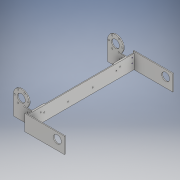
# Autodesk Inventor part: Pivot Bracket 2
Saved by Autodesk Inventor 2017 (Build 210142000, 142)
## iProperties
Created: 2017-06-10
Part Number: Pivot Bracket 2
Material: Generic
Document SubType Name: Modeling
Designer: Matthew
Density: 1 g/cm^3
Appearance: Aluminum - Polished
Author: Matthew
Autodesk Inventor part; units mm, degrees
ref_plane "YZ Plane" through (0, 0, 0) normal (1, 0, 0) x (0, 1, 0)
ref_plane "XZ Plane" through (0, 0, 0) normal (0, 1, 0) x (-1, 0, 0)
ref_plane "XY Plane" through (0, 0, 0) normal (0, 0, 1) x (1, 0, 0)
sketch "Sketch1" plane through (0, 0, 0) normal (0, 1, 0) x (-1, 0, 0)
  line L0 (0, 0) -> (-88.9, 0)
  line L1 (-88.9, 0) -> (-88.9, -3.175)
  line L2 (-88.9, -3.175) -> (0, -3.175)
  line L3 (0, -3.175) -> (0, 0)
  dimension "d0" = 88.9
  dimension "d1" = 3.175
  constraints: 8 end point, 2 parallel, 1 horizontal, 1 perpendicular
  measures "d0" distance of L2.end L1.end
  measures "d1" distance of L1.end L0.end
extrude "Extrusion1" add sketch "Sketch1" along normal blind 25.4
sketch "Sketch2" plane through (0, 0, 0) normal (0, 0, 1) x (1, 0, 0)
  line L0 (88.9, 0) -> (88.9, 25.4) projected
  circle A0 centre (88.9, 12.7) radius 3.175
  point P0 (0, 0)
  dimension "d4" = 6.35
  constraints: 1 centre point, 1 midpoint
  measures "d4" diameter of A0
extrude "Extrusion2" cut sketch "Sketch2" against normal blind 25.4
sketch "Sketch3" plane through (0, 0, 0) normal (0, 0, 1) x (1, 0, 0)
  arc A0 (88.9, 15.875) -> (88.9, 9.525) centre (88.9, 12.7) ccw projected
  line L0 (88.9, 25.4) -> (0, 25.4) projected
  circle A1 centre (88.9, 12.7) radius 12.7
  line L1 (88.9, 15.875) -> (88.9, 25.4) projected
  circle A2 centre (88.9, 12.7) radius 3.175
  point P0 (0, 0)
  constraints: 2 coincident, 2 vertical alignment, 4 other
extrude "Extrusion3" add sketch "Sketch3" against normal blind 3.175
sketch "Sketch4" plane through (0, 0, -3.175) normal (-1, 0, 0) x (0, 0, 1)
  line L0 (0, 0) -> (0, 25.4) projected
  line L1 (0, 0) -> (53.975, 0)
  line L2 (53.975, 0) -> (53.975, 25.4)
  line L3 (53.975, 25.4) -> (0, 25.4)
  line L4 (0, 25.4) -> (0, 0)
  point P0 (3.175, 0)
  dimension "d9" = 53.975
  constraints: 8 end point, 2 parallel, 1 horizontal, 1 perpendicular
  measures "d9" distance of L3.end L2.end
extrude "Extrusion4" add sketch "Sketch4" against normal blind 3.175
sketch "Sketch5" plane through (3.175, 0, -3.175) normal (1, 0, 0) x (0, 0, -1)
  line L0 (-3.175, 25.4) -> (-53.975, 25.4) projected
  line L1 (-3.175, 25.4) -> (-53.975, 12.7)
  line L2 (-53.975, 12.7) -> (-53.975, -12.7)
  line L3 (-53.975, 25.4) -> (-53.975, 0) projected
  line L4 (-53.975, -12.7) -> (-3.175, 0)
  line L5 (-3.175, 25.4) -> (-3.175, 0) projected
  line L6 (-3.175, 25.4) -> (-3.175, 0)
  dimension "d12" = 12.7
  dimension "d13" = 25.4
  constraints: 8 end point, 3 equal length, 1 point on line, 1 vertical alignment
  measures "d12" distance of L0.end L1.end
  measures "d13" distance of L1.end L2.end
sketch "Sketch6" plane through (3.175, 0, -3.175) normal (1, 0, 0) x (0, 0, -1)
  line L0 (-3.175, 25.4) -> (-3.175, 0) projected
  line L1 (-3.175, 25.4) -> (-53.975, 25.4) projected
  line L2 (-53.975, 25.4) -> (-53.975, 0) projected
  line L3 (-53.975, 0) -> (-3.175, 0) projected
extrude "Extrusion5" cut sketch "Sketch6" against normal blind 25.4
extrude "Extrusion6" add sketch "Sketch5" against normal blind 3.175 contours L5 L4 L2 L1
mirror "Mirror3" about plane through (88.9, 0, -3.175) normal (0, 0, -1)
sketch "Sketch8" plane through (0, -12.7, 50.8) normal (-1, 0, 0) x (0, 0, 1)
  line L0 (-250.825, 44.45) -> (142.875, 44.45)
  line L1 (142.875, 44.45) -> (142.875, -6.35)
  line L2 (142.875, -6.35) -> (-250.825, -6.35)
  line L3 (-250.825, -6.35) -> (-250.825, 44.45)
  line L4 (-50.8, 12.7) -> (0, 0) construction
  line L5 (-107.95, 38.1) -> (0, 38.1) construction
  line L6 (0, 38.1) -> (0, 0) construction
  line L7 (0, 0) -> (-107.95, 0) construction
  line L8 (-107.95, 0) -> (-107.95, 38.1) construction
  point P0 (-53.975, 44.45)
  point P1 (-250.825, 19.05)
  point P2 (-53.975, 38.1)
  point P3 (0, 19.05)
  dimension "d20" = 393.7
  dimension "d21" = 50.8
  dimension "d22" = 53.975
  dimension "d23" = 19.05
  constraints: 16 end point, 4 midpoint, 4 parallel, 2 horizontal, 2 perpendicular, 1 horizontal alignment, 1 vertical alignment
  measures "d20" distance of L1.end L2.end
  measures "d21" distance of L0.end L1.end
  measures "d22" distance from line of L6 point (-53.975, 38.1)
  measures "d23" distance from line of L7 point (0, 19.05)
extrude "Extrusion8" add sketch "Sketch8" against normal blind 3.175
sketch "Sketch9" plane through (0, -19.05, -200.025) normal (-1, 0, 0) x (0, 0, 1)
  line L0 (0, 0) -> (0, 50.8) projected
  line L1 (393.7, 0) -> (0, 0) projected
  line L2 (0, 50.8) -> (3.175, 50.8)
  line L3 (3.175, 50.8) -> (3.175, 0)
  line L4 (3.175, 0) -> (0, 0)
  line L5 (0, 0) -> (0, 50.8)
  line L6 (0, 50.8) -> (393.7, 50.8) projected
  line L7 (393.7, 50.8) -> (390.525, 50.8)
  line L8 (390.525, 50.8) -> (390.525, 0)
  line L9 (390.525, 0) -> (393.7, 0)
  line L10 (393.7, 0) -> (393.7, 50.8)
  point P0 (200.025, 19.05)
  dimension "d26" = 3.175
  dimension "d27" = 3.175
  constraints: 16 end point, 4 parallel, 2 horizontal, 2 perpendicular, 2 point on line
  measures "d26" distance of L3.end L4.end
  measures "d27" distance of L9.end L8.end
extrude "Extrusion9" add sketch "Sketch9" along normal blind 139.7 contours L0 L2 L3 L1 | L8 L6 L10 L1
sketch "Sketch10" plane through (0, -19.05, -196.85) normal (-1, 0, 0) x (0, 0, 1)
  line L0 (387.35, 0) -> (0, 0) projected
  ellipse E0 centre (12.7, 0) end of major axis (12.7, 19.05) minor radius 9.525
  line L1 (0, 0) -> (0, 50.8) projected
  ellipse E1 centre (12.7, 63.5) end of major axis (12.7, 44.45) minor radius 9.525
  line L2 (0, 50.8) -> (387.35, 50.8) projected
  point P0 (196.85, 19.05)
  dimension "d30" = 19.05
  dimension "d31" = 9.525
  dimension "d33" = 19.05
  dimension "d34" = 9.525
  dimension "d32" = 12.7
  dimension "d35" = 12.7
  constraints: 1 horizontal, 1 point on line, 1 vertical alignment, 4 other
  measures "d32" distance from line of point (12.7, 0) L1
  measures "d35" distance from line of L2 point (12.7, 63.5)
extrude "Extrusion10" cut sketch "Sketch10" against normal blind 139.7
sketch "Sketch11" plane through (3.175, -19.05, 193.675) normal (0, 0, 1) x (1, 0, 0)
  circle A0 centre (-117.475, 34.925) radius 14.2875
  line L0 (-142.875, 0) -> (-142.875, 50.8) projected
  line L1 (-142.875, 50.8) -> (0, 50.8) projected
  point P0 (-3.175, 19.05)
  dimension "d38" = 28.575
  dimension "d39" = 25.4
  dimension "d40" = 15.875
  constraints: 1 centre point
  measures "d38" diameter of A0
  measures "d39" distance from line of L0 A0.centre
  measures "d40" distance from line of A0.centre L1
extrude "Extrusion11" cut sketch "Sketch11" against normal blind 395.2875
ref_plane "Work Plane1" through (3.175, -19.05, 168.275) normal (0, 0, 1) x (1, 0, 0)
sketch "Sketch12" plane through (3.175, -19.05, 168.275) normal (0, 0, 1) x (1, 0, 0)
  line L0 (0, 44.45) -> (0, 19.05) projected
  line L1 (0, 19.05) -> (85.725, 19.05) projected
  arc A0 (85.725, 19.05) -> (85.725, 44.45) centre (85.725, 31.75) ccw projected
  line L2 (0, 44.45) -> (85.725, 44.45) projected
  circle A1 centre (85.725, 31.75) radius 3.175 projected
  point P0 (-3.175, 19.05)
extrude "Extrusion12" add sketch "Sketch12" against normal blind 3.175
ref_plane "Work Plane2" through (3.175, -19.05, -3.175) normal (0, 0, 1) x (1, 0, 0)
sketch "Sketch13" plane through (88.9, 12.7, -6.35) normal (0, 0, -1) x (-1, 0, 0)
  line L0 (85.725, 12.7) -> (85.725, -12.7) projected
  line L1 (85.725, 12.7) -> (0, 12.7) projected
  arc A0 (0, 12.7) -> (0, -12.7) centre (0, 0) ccw projected
  line L2 (85.725, -12.7) -> (0, -12.7) projected
  circle A1 centre (0, 0) radius 3.175 projected
  point P0 (88.9, -12.7)
extrude "Extrusion13" cut sketch "Sketch13" against normal blind 6.35
mirror "Mirror4" about plane through (3.175, -19.05, -3.175) normal (0, 0, 1) of "Extrusion12"
sketch "Sketch15" plane through (3.175, 0, -3.175) normal (1, 0, 0) x (0, 0, -1)
  line L0 (-196.85, 31.75) -> (-196.85, -19.05) projected
  line L1 (196.85, -19.05) -> (196.85, 31.75) projected
  line L2 (-196.85, -19.05) -> (-196.85, 31.75) projected
  line L3 (173.8755, 31.75) -> (-196.85, 31.75) projected
  circle A0 centre (-44.45, 0) radius 2.032
  circle A1 centre (44.45, 0) radius 2.032
  point P0 (-3.175, 0)
  dimension "d51" = 152.4
  dimension "d52" = 152.4
  dimension "d54" = 31.75
  dimension "d63" = 4.064
  dimension "d64" = 4.064
  constraints: 2 centre point, 2 coincident, 1 horizontal alignment
  measures "d51" distance from line of L0 point (-44.45, 0)
  measures "d52" distance from line of L1 point (44.45, 0)
  measures "d54" distance from line of L3 point (-44.45, 0)
  measures "d63" diameter of A0
  measures "d64" diameter of A1
sketch "Sketch16" plane through (3.175, 0, -3.175) normal (1, 0, 0) x (0, 0, -1)
  line L0 (-171.45, 25.4) -> (-168.275, 25.4) projected
  line L1 (-168.275, 0) -> (-168.275, 25.4) projected
  line L2 (-171.45, 0) -> (-168.275, 0) projected
  line L3 (-168.275, 0) -> (0, 0)
  line L4 (0, 0) -> (0, 31.75)
  line L5 (173.8755, 31.75) -> (-193.675, 31.75) projected
  circle A0 centre (-142.875, 15.875) radius 2.032
  circle A1 centre (-130.175, 9.525) radius 2.032
  circle A2 centre (142.875, 15.875) radius 2.032
  circle A3 centre (130.175, 9.525) radius 2.032
  point P0 (-3.175, 0)
  dimension "d53" = 9.525
  dimension "d55" = 25.4
  dimension "d56" = 38.1
  dimension "d57" = 9.525
  dimension "d58" = 168.275
  dimension "d59" = 4.064
  dimension "d60" = 4.064
  constraints: 4 centre point, 4 coincident, 4 end point, 4 symmetric about line, 1 horizontal, 1 point on line, 1 vertical, 2 other
  measures "d53" distance from line of L0 point (-142.875, 15.875)
  measures "d55" distance from line of L1 point (-142.875, 15.875)
  measures "d56" distance from line of L1 point (-130.175, 9.525)
  measures "d57" distance from line of L2 point (-130.175, 9.525)
  measures "d58" distance of L1.start L3.end
  measures "d59" diameter of A0
  measures "d60" diameter of A1
extrude "Extrusion14" cut sketch "Sketch16" against normal blind 6.35
extrude "Extrusion15" cut sketch "Sketch15" against normal blind 6.35
sketch "Sketch17" plane through (3.175, 0, -3.175) normal (1, 0, 0) x (0, 0, -1)
  circle A0 centre (187.325, 21.4313) radius 1.5875
  circle A1 centre (187.325, 3.9688) radius 1.5875
  line L0 (171.45, 25.4) -> (171.45, 0) projected
  line L1 (171.45, 25.4) -> (168.275, 25.4) projected
  line L2 (-168.275, 25.4) -> (-168.275, 0) projected
  line L3 (-168.275, 0) -> (0, 0)
  line L4 (168.275, 0) -> (168.275, 25.4) projected
  line L5 (0, 0) -> (0, 31.75)
  line L6 (173.8755, 31.75) -> (-193.675, 31.75) projected
  circle A2 centre (-187.325, 21.4313) radius 1.5875
  circle A3 centre (-187.325, 3.9688) radius 1.5875
  point P0 (-3.175, 0)
  dimension "d67" = 3.175
  dimension "d68" = 3.175
  dimension "d69" = 15.875
  dimension "d70" = 17.4625
  dimension "d71" = 3.9688
  dimension "d72" = 168.275
  constraints: 4 centre point, 4 end point, 2 symmetric about line, 1 perpendicular, 1 point on line, 1 vertical, 1 vertical alignment, 2 other
  measures "d67" diameter of A0
  measures "d68" diameter of A1
  measures "d69" distance from line of L0 A0.centre
  measures "d70" distance of A1.centre A0.centre
  measures "d71" distance from line of L1 A0.centre
  measures "d72" distance of L2.end L3.end
extrude "Extrusion16" cut sketch "Sketch17" against normal blind 6.35
sketch "Sketch18" plane through (3.175, 0, -3.175) normal (1, 0, 0) x (0, 0, -1)
  circle A0 centre (-187.325, 21.4313) radius 1.5875 projected
  circle A1 centre (-187.325, 3.9688) radius 1.5875 projected
  circle A2 centre (-142.875, 15.875) radius 2.032 projected
  circle A3 centre (-130.175, 9.525) radius 2.032 projected
  circle A4 centre (-44.45, 0) radius 2.032 projected
  circle A5 centre (44.45, 0) radius 2.032 projected
  circle A6 centre (130.175, 9.525) radius 2.032 projected
  circle A7 centre (142.875, 15.875) radius 2.032 projected
  circle A8 centre (187.325, 21.4313) radius 1.5875 projected
  circle A9 centre (187.325, 3.9688) radius 1.5875 projected
  line L0 (-196.85, 31.75) -> (-196.85, -19.05) projected
  line L1 (173.8755, 31.75) -> (-196.85, 31.75) projected
  point P0 (-3.175, 0)
  dimension "d75" = 9.525
  dimension "d76" = 53.975
  dimension "d77" = 66.675
  dimension "d78" = 152.4
  dimension "d79" = 10.3187
  dimension "d80" = 27.7812
  dimension "d81" = 15.875
  dimension "d82" = 22.225
  dimension "d83" = 31.75
  measures "d75" distance from line of L0 A1.centre
  measures "d76" distance from line of A2.centre L0
  measures "d77" distance from line of L0 A3.centre
  measures "d78" distance from line of L0 A4.centre
  measures "d79" distance from line of A0.centre L1
  measures "d80" distance from line of A1.centre L1
  measures "d81" distance from line of L1 A2.centre
  measures "d82" distance from line of A3.centre L1
  measures "d83" distance from line of A4.centre L1
sketch "Sketch19" plane through (88.9, 25.4, -174.625) normal (0, 0, -1) x (-1, 0, 0)
  circle A0 centre (69.85, -4.7625) radius 1.5875
  circle A1 centre (61.9125, -12.7) radius 1.5875
  circle A2 centre (69.85, -20.6375) radius 1.5875
  circle A3 centre (77.7875, -12.7) radius 1.5875
  line L0 (85.725, 0) -> (85.725, -25.4) projected
  circle A4 centre (0, -12.7) radius 3.175 projected
  point P0 (88.9, -25.4)
  dimension "d84" = 3.175
  dimension "d85" = 3.175
  dimension "d86" = 3.175
  dimension "d87" = 3.175
  dimension "d88" = 15.875
  dimension "d89" = 7.9375
  dimension "d90" = 15.875
  dimension "d91" = 15.875
  dimension "d92" = 7.9375
  constraints: 4 centre point, 2 horizontal alignment, 1 coincident, 1 vertical alignment
  measures "d84" diameter of A0
  measures "d85" diameter of A1
  measures "d86" diameter of A2
  measures "d87" diameter of A3
  measures "d88" distance from line of L0 A0.centre
  measures "d89" distance from line of L0 A3.centre
  measures "d90" distance of A3.centre A1.centre
  measures "d91" distance of A2.centre A0.centre
  measures "d92" vertical distance of A4.centre A0.centre
extrude "Extrusion17" cut sketch "Sketch19" against normal blind 390.525 contours A0 | A1 | A2 | A3
sketch "Sketch20" plane through (3.175, 0, -3.175) normal (1, 0, 0) x (0, 0, -1)
  line L0 (-168.275, 25.4) -> (-168.275, 0) projected
  line L1 (-168.275, 0) -> (0, 0)
  line L2 (168.275, 0) -> (168.275, 25.4) projected
  line L3 (0, 0) -> (0, 31.75)
  line L4 (173.8755, 31.75) -> (-193.675, 31.75) projected
  point P0 (-3.175, 0)
  dimension "d95" = 168.275
  constraints: 4 end point, 2 perpendicular, 1 point on line
  measures "d95" distance of L0.end L1.end
sketch "Sketch21" plane through (88.9, 25.4, -174.625) normal (0, 0, -1) x (-1, 0, 0)
  circle A0 centre (0, -12.7) radius 3.175 projected
  circle A1 centre (0, -12.7) radius 28.575
  point P0 (88.9, -25.4)
  dimension "d96" = 57.15
  constraints: 1 centre point, 1 coincident
  measures "d96" diameter of A1
extrude "Extrusion18" add sketch "Sketch21" against normal up to surface (3.175 mm away)
sketch "Sketch22" plane through (3.175, 0, -174.625) normal (0, 0, -1) x (-1, 0, 0)
  line L0 (0, 31.75) -> (142.875, 31.75) projected
  line L1 (0, 31.75) -> (-64.4265, 31.75)
  arc A0 (-60.1273, 25.4) -> (-60.1273, 0) centre (-85.725, 12.7) ccw projected
  line L2 (-85.725, -15.875) -> (0, -15.875)
  line L3 (0, 31.75) -> (0, -19.05) projected
  line L4 (-64.4265, 31.75) -> (-85.725, -15.875)
  line L5 (-22.4352, 23.7734) -> (-32.2132, 12.7)
  line L6 (-32.2132, 12.7) -> (-15.4548, 1.4363)
  line L7 (-15.4548, 1.4363) -> (-2.7633, 13.4933)
  line L8 (-2.7633, 13.4933) -> (-14.4053, 23.7734)
  line L9 (-14.4053, 23.7734) -> (-22.4352, 23.7734)
  line L10 (0, 25.4) -> (0, 0) projected
  line L11 (0, 31.75) -> (0, -15.875)
  point P0 (3.175, 0)
  constraints: 18 end point, 3 perpendicular, 2 horizontal, 2 point on circle, 1 point on line, 1 vertical alignment
extrude "Extrusion19" add sketch "Sketch22" against normal blind 3.175 contours L3 L2 L4 L1
sketch "Sketch23" plane through (67.6015, 31.75, -174.625) normal (0, 0, -1) x (-1, 0, 0)
  circle A0 centre (-21.2985, -19.05) radius 28.321
  circle A1 centre (-33.2048, 1.5722) radius 2.5908
  circle A2 centre (2.514, -19.05) radius 2.5908
  circle A3 centre (-33.2048, -39.6722) radius 2.5908
  circle A4 centre (-21.2985, -19.05) radius 14.2875
  circle A5 centre (-9.3923, -39.6722) radius 2.5908
  circle A6 centre (-9.3923, 1.5722) radius 2.5908
  circle A7 centre (-45.111, -19.05) radius 2.5908
  circle A8 centre (-21.2985, -19.05) radius 3.175 projected
  point P0 (67.6015, -31.75)
  dimension "d101" = 56.642
  dimension "d102" = 28.575
  dimension "d103" = 11.9062
  dimension "d104" = 20.6222
  dimension "d105" = 23.8125
  dimension "d106" = 23.8125
  dimension "d107" = 41.2445
  dimension "d108" = 23.8125
  constraints: 8 centre point, 4 horizontal alignment, 2 vertical alignment, 1 coincident, 1 concentric
  measures "d101" diameter of A0
  measures "d102" diameter of A4
  measures "d103" horizontal distance of A0.centre A6.centre
  measures "d104" vertical distance of A0.centre A6.centre
  measures "d105" distance of A0.centre A2.centre
  measures "d106" distance of A1.centre A6.centre
  measures "d107" distance of A5.centre A6.centre
  measures "d108" distance of A0.centre A7.centre
extrude "Extrusion20" cut sketch "Sketch23" against normal blind 3.175 contours A1 | A2 | A3 | A5 | A6 | A7
sketch "Sketch24" plane through (67.6015, 31.75, -174.625) normal (0, 0, -1) x (-1, 0, 0)
  arc A0 (0, 0) -> (-21.2985, -47.625) centre (-21.2985, -19.05) ccw projected
  line L0 (-21.2985, 9.525) -> (0, 9.525)
  line L1 (0, 0) -> (64.4265, 0) projected
  line L2 (0, 9.525) -> (0, 0)
  arc A1 (0, 0) -> (-21.2985, 9.525) centre (-21.2985, -19.05) ccw
  point P0 (67.6015, -31.75)
  constraints: 4 end point, 3 point on circle, 1 centre point, 1 concentric, 1 horizontal, 1 perpendicular, 1 tangent
extrude "Extrusion21" add sketch "Sketch24" against normal blind 3.175
sketch "Sketch25" plane through (88.9, -15.875, -174.625) normal (0, 0, -1) x (-1, 0, 0)
  circle A0 centre (0, 28.575) radius 3.175 projected
  circle A1 centre (0, 28.575) radius 14.2875
  point P0 (88.9, 15.875)
  dimension "d113" = 28.575
  constraints: 1 centre point, 1 coincident
  measures "d113" diameter of A1
extrude "Extrusion22" cut sketch "Sketch25" against normal blind 3.175
sketch "Sketch26" plane through (3.175, 0, -3.175) normal (1, 0, 0) x (0, 0, -1)
  line L0 (168.275, 31.75) -> (-196.85, 31.75) projected
  line L1 (168.275, 31.75) -> (123.825, 31.75)
  line L2 (123.825, 31.75) -> (123.825, 0)
  line L3 (123.825, 0) -> (168.275, 0)
  line L4 (168.275, 0) -> (168.275, 31.75)
  circle A0 centre (130.175, 9.525) radius 2.032 projected
  circle A1 centre (142.875, 15.875) radius 2.032 projected
  point P0 (-3.175, 0)
  dimension "d116" = 44.45
  dimension "d117" = 31.75
  constraints: 8 end point, 3 perpendicular, 1 point on line
  measures "d116" distance of L0.start L1.end
  measures "d117" distance of L1.end L2.end
extrude "Extrusion23" add sketch "Sketch26" along normal blind 3.175
mirror "Mirror5" about plane through (3.175, -19.05, -3.175) normal (0, 0, 1) of "Extrusion12", "Mirror4", "Extrusion22", "Extrusion20", "Extrusion18", "Extrusion21", "Extrusion19", "Extrusion23", "Extrusion17"
sketch "Sketch27" plane through (88.9, -15.875, -174.625) normal (0, 0, -1) x (-1, 0, 0)
  circle A0 centre (0, 28.575) radius 14.2875 projected
  point P0 (88.9, 15.875)
extrude "Extrusion24" cut sketch "Sketch27" against normal blind 3.175
sketch "Sketch28" plane through (3.175, -19.05, -200.025) normal (0, 0, -1) x (-1, 0, 0)
  line L0 (0, 50.8) -> (142.875, 50.8) projected
  line L1 (0, 50.8) -> (142.875, 50.8)
  line L2 (142.875, 50.8) -> (142.875, 57.15)
  line L3 (142.875, 57.15) -> (0, 57.15)
  line L4 (0, 57.15) -> (0, 50.8)
  point P0 (3.175, 19.05)
  dimension "d122" = 6.35
  constraints: 8 end point, 2 parallel, 1 horizontal, 1 perpendicular
  measures "d122" distance of L2.end L1.end
extrude "Extrusion25" add sketch "Sketch28" against normal blind 3.175
mirror "Mirror6" about plane through (3.175, -19.05, -3.175) normal (0, 0, 1) of "Extrusion25"
extrude "Extrusion26" cut sketch "Sketch23" against normal blind 519.1125 contours A2
sketch "Sketch29" plane through (88.9, -15.875, -174.625) normal (0, 0, -1) x (-1, 0, 0)
  circle A0 centre (0, 28.575) radius 14.2875 projected
  circle A1 centre (-11.9063, 49.1972) radius 2.5908 projected
  circle A2 centre (11.9062, 49.1972) radius 2.5908 projected
  circle A3 centre (23.8125, 28.575) radius 2.5908 projected
  circle A4 centre (11.9062, 7.9528) radius 2.5908 projected
  circle A5 centre (-11.9063, 7.9528) radius 2.5908 projected
  circle A6 centre (-23.8125, 28.575) radius 2.5908 projected
  circle A7 centre (47.625, 69.85) radius 14.2875
  circle A8 centre (35.7187, 90.4722) radius 2.5908
  circle A9 centre (59.5312, 90.4722) radius 2.5908
  circle A10 centre (71.4375, 69.85) radius 2.5908
  circle A11 centre (59.5312, 49.2278) radius 2.5908
  circle A12 centre (35.7187, 49.2278) radius 2.5908
  circle A13 centre (23.8125, 69.85) radius 2.5908
  circle A14 centre (47.625, 69.85) radius 28.575
  point P0 (88.9, 15.875)
  dimension "d127" = 41.275
  dimension "d128" = 41.275
  dimension "d129" = 41.275
  dimension "d130" = 41.275
  dimension "d131" = 41.275
  dimension "d132" = 41.275
  dimension "d133" = 41.275
  dimension "d134" = 47.625
  dimension "d135" = 47.625
  dimension "d136" = 47.625
  dimension "d137" = 47.625
  dimension "d138" = 47.625
  dimension "d139" = 47.625
  dimension "d140" = 47.625
  dimension "d141" = 57.15
  constraints: 8 centre point, 1 coincident
  measures "d127" vertical distance of A1.centre A8.centre
  measures "d128" vertical distance of A13.centre A6.centre
  measures "d129" vertical distance of A9.centre A2.centre
  measures "d130" vertical distance of A3.centre A10.centre
  measures "d131" vertical distance of A11.centre A4.centre
  measures "d132" vertical distance of A5.centre A12.centre
  measures "d133" vertical distance of A0.centre A7.centre
  measures "d134" horizontal distance of A0.centre A7.centre
  measures "d135" horizontal distance of A2.centre A9.centre
  measures "d136" horizontal distance of A3.centre A10.centre
  measures "d137" horizontal distance of A11.centre A4.centre
  measures "d138" horizontal distance of A12.centre A5.centre
  measures "d139" horizontal distance of A13.centre A6.centre
  measures "d140" horizontal distance of A1.centre A8.centre
  measures "d141" diameter of A14
sketch "Sketch30" plane through (88.9, -15.875, -174.625) normal (0, 0, -1) x (-1, 0, 0)
  line L0 (-36.1671, 81.9483) -> (-25.1444, 2.22)
  line L1 (-25.1444, 2.22) -> (19.05, 13.7583)
  circle A0 centre (47.625, 69.85) radius 28.575 projected
  line L2 (19.05, 13.7583) -> (19.05, 69.85)
  line L3 (68.9235, 50.8) -> (85.725, 50.8)
  line L4 (85.725, 47.625) -> (85.725, 53.975) projected
  line L5 (85.725, 50.8) -> (48.9227, 121.8375)
  line L6 (48.9227, 121.8375) -> (-36.1671, 81.9483)
  point P0 (88.9, 15.875)
  constraints: 12 end point, 2 point on circle, 1 midpoint, 1 tangent, 1 vertical
extrude "Extrusion27" cut sketch "Sketch30" against normal blind 519.1125 contours L6 L5 A0 L2 L1 L0 | L5 L3 A0
extrude "Extrusion28" cut sketch "Sketch29" against normal blind 519.1125 contours A8 | A9 | A10 | A11 | A12 | A13
extrude "Extrusion29" add sketch "Sketch29" against normal blind 3.175 contours A14
mirror "Mirror7" about plane through (3.175, -19.05, -3.175) normal (0, 0, 1)
sketch "Sketch34" plane through (69.85, -15.875, -174.625) normal (0, 0, -1) x (-1, 0, 0)
  arc A0 (7.3533, 69.85) -> (19.2595, 49.2278) centre (28.575, 69.85) ccw projected
  circle A1 centre (28.575, 69.85) radius 26.2298
  circle A2 centre (50.8, 20.6375) radius 1.5875 projected
  circle A3 centre (58.7375, 28.575) radius 1.5875 projected
  line L0 (58.7375, 28.575) -> (45.1684, 28.575)
  circle A4 centre (50.8, 36.5125) radius 1.5875
  point P0 (69.85, 15.875)
  point P1 (14.6447, 47.625)
  point P2 (42.5053, 47.625)
  constraints: 2 end point, 1 centre point, 1 coincident, 1 horizontal, 1 symmetric about line, 5 other
extrude "Extrusion33" cut sketch "Sketch34" against normal blind 385.7625 contours A1 | A4
extrude "Extrusion34" add sketch "Sketch29" against normal blind 3.175 contours A14
sketch "Sketch35" plane through (88.9, -15.875, -174.625) normal (0, 0, -1) x (-1, 0, 0)
  line L0 (-57.6363, 49.8409) -> (12.379, -45.4409)
  arc A0 (25.1644, -24.4363) -> (12.379, -45.4409) centre (23.0923, -37.5685) ccw
  line L1 (25.1644, -24.4363) -> (19.05, -16.1153)
  line L2 (19.05, 57.15) -> (19.05, 13.7583) projected
  line L3 (19.05, -16.1153) -> (19.05, 57.15)
  line L4 (19.05, 57.15) -> (-60.0716, 96.4163)
  line L5 (-60.0716, 96.4163) -> (-57.6363, 49.8409)
  point P0 (88.9, 15.875)
  constraints: 10 end point, 2 point on circle, 1 centre point, 1 tangent, 1 vertical, 1 vertical alignment
extrude "Extrusion35" cut sketch "Sketch35" against normal blind 3.175
sketch "Sketch36" plane through (3.175, -15.875, -174.625) normal (0, 0, -1) x (-1, 0, 0)
  arc A0 (-20.1395, 47.625) -> (-56.0605, 47.625) centre (-38.1, 69.85) ccw projected
  line L0 (-66.675, 69.85) -> (-66.675, 21.0483)
  line L1 (-66.675, 21.0483) -> (-42.1468, 25.1812)
  line L2 (-42.1468, 25.1812) -> (-20.1395, 47.625)
  line L3 (-56.0605, 47.625) -> (-64.4265, 47.625) projected
  line L4 (-56.0605, 47.625) -> (-42.1468, 25.1812)
  point P0 (3.175, 15.875)
  constraints: 8 end point, 1 point on circle, 1 tangent, 1 vertical
extrude "Extrusion36" add sketch "Sketch36" against normal blind 3.175 contours A0 L4 L1 L0
mirror "Mirror8" about plane through (3.175, -19.05, -3.175) normal (0, 0, 1)
sketch "Sketch37" plane through (3.175, -15.875, -174.625) normal (0, 0, -1) x (-1, 0, 0)
  line L0 (-66.675, 13.7583) -> (-66.675, 69.85) projected
  line L1 (-66.675, 61.542) -> (-125.4832, 61.542)
  line L2 (-125.4832, 61.542) -> (-125.4832, -13.7943)
  line L3 (-125.4832, -13.7943) -> (-66.675, -13.7943)
  line L4 (-66.675, -13.7943) -> (-66.675, 61.542)
  point P0 (3.175, 15.875)
  constraints: 8 end point, 2 parallel, 1 horizontal, 1 perpendicular, 1 point on line
extrude "Extrusion37" cut sketch "Sketch37" against normal blind 442.9125
body "Solid1"
